# Autodesk Inventor part: soporteDerecho
Saved by Autodesk Inventor 2015 (Build 190159000, 159)
## iProperties
Created: 2015-02-22
Part Number: soporteDerecho
Material: Genérico
Document SubType Name: Modeling
Designer: jorge
Density: 1 g/cm^3
Appearance: Valor por defecto
Author: jorge
Autodesk Inventor part; units mm, degrees
note: some values were not read from the file. Chosen so that the rebuilt part matches the saved one: direction of "Agujero1"; direction of "Agujero2".
ref_plane "YZ Plane" through (0, 0, 0) normal (1, 0, 0) x (0, 1, 0)
ref_plane "XZ Plane" through (0, 0, 0) normal (0, 1, 0) x (-1, 0, 0)
ref_plane "Plano de trabajo1" through (64.5, -49.5, 12.8) normal (0, 0, 1) x (1, 0, 0)
sketch "Boceto1" plane through (0, 0, 0) normal (0, 0, 1) x (1, 0, 0)
  line L0 (-63.5, 34.5) -> (63.5, 34.5)
  line L1 (63.5, -34.5) -> (-63.5, -34.5)
  line L2 (63.5, 34.5) -> (63.5, -34.5)
  line L3 (64.5, -16.5586) -> (64.5, -23.5586)
  line L4 (64.5, -23.5586) -> (64.5, -44.5)
  line L5 (64.5, -49.5) -> (64.5, -23.5586)
  line L6 (64.5, -16.5586) -> (64.5, -23.5586)
  line L7 (63.5, -34.5) -> (57.5, -34.5)
  line L8 (57.5, -34.5) -> (57.5, -9.5)
  line L9 (57.5, -9.5) -> (63.5, -9.5)
  line L10 (63.5, -9.5) -> (63.5, -34.5)
  point P0 (0, 0)
extrude "Extrusión1" add sketch "Boceto1" along normal up to surface (12.8 mm away)
sketch "Boceto2" plane through (57.5, -34.5, 0) normal (-1, 0, 0) x (0, 0, 1)
  line L0 (0, 0) -> (3, 0)
  line L1 (0, 25) -> (3, 25)
  line L2 (0, 25) -> (12.8, 25) projected
  line L3 (12.8, 0) -> (12.8, 25) projected
  arc A0 (12.8, 10.9414) -> (-1.2, 10.9414) centre (5.8, 10.9414) ccw projected
  arc A1 (12.8, 18.0828) -> (3, 20.5414) centre (5.8, 10.9414) ccw
  line L4 (3, 25) -> (3, 20.5414)
  line L5 (12.8, 0) -> (12.8, 5)
  line L6 (3, 1.3414) -> (3, 0)
  line L7 (3, 0) -> (12.8, 0)
  arc A2 (3, 1.3414) -> (12.8, 3.8) centre (5.8, 10.9414) ccw
  point P0 (0, 34.5)
  dimension "d4" = 3
  dimension "d6" = 3
  dimension "d8" = 3
  dimension "d9" = 5
  constraints: 12 end point, 4 point on circle, 4 point on line, 2 centre point, 2 horizontal, 1 coincident, 1 vertical
  measures "d4" distance of L0.start L0.end
  measures "d6" distance of L1.start L1.end
  measures "d8" radial gap between concentric circles of A0 A1
  measures "d9" distance of L3.start L5.end
extrude "Extrusión2" cut sketch "Boceto2" against normal up to surface (6 mm away)
hole "Agujero1" at (57.5, -23.5586, 5.8) direction (1, 0, 0) diameter 9 end up to surface
sketch "Boceto3" plane through (57.5, -34.5, 3) normal (0, 0, 1) x (1, 0, 0)
  line L0 (0, 5) -> (6, 5) projected
  line L1 (6, 0) -> (0, 0) projected
  line L2 (6, 25) -> (6, 20.5414) projected
  line L3 (0, 25) -> (6, 25) projected
  line L4 (0, 20.5414) -> (0, 25) projected
  line L5 (0, 20.5414) -> (6, 20.5414) projected
  line L6 (6, 5) -> (0, 0)
  line L7 (0, 20.5414) -> (6, 25)
  point P0 (-57.5, 34.5)
  point P1 (3, 22.7707)
  point P2 (3, 2.5)
  constraints: 4 end point, 2 midpoint
hole "Agujero2" at (60.5, -11.7293, 3) at (60.5, -32, 3) direction (0, 0, -1) diameter 2.5 end up to surface
sketch "Boceto4" plane through (57.5, -16.4172, 12.8) normal (0, 0, 1) x (1, 0, 0)
  arc A0 (2.5308, -16.7414) -> (3.4692, -16.7414) centre (3, -15.5828) ccw projected
  circle A1 centre (3, -15.5828) radius 2
  point P0 (-57.5, 16.4172)
  dimension "d30" = 4
  constraints: 1 centre point, 1 coincident
  measures "d30" diameter of A1
extrude "Extrusión3" cut sketch "Boceto4" against normal up to surface (9.8 mm away)
